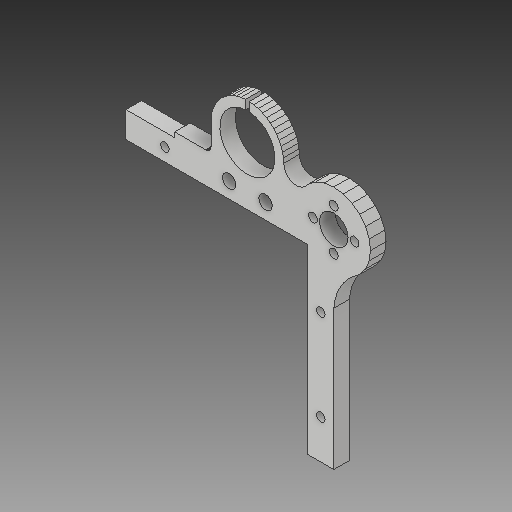
# Autodesk Inventor part: Left Bed Holder Mid
Saved by Autodesk Inventor 2017 (Build 210142000, 142)
## iProperties
Created: 2016-07-12
Part Number: Left Bed Holder Mid
Material: Generic
Document SubType Name: Modeling
Designer: joshmamo
Density: 1 g/cm^3
Appearance: Default
Author: joshmamo
Autodesk Inventor part; units mm, degrees
ref_plane "YZ Plane" through (0, 0, 0) normal (1, 0, 0) x (0, 1, 0)
ref_plane "XZ Plane" through (0, 0, 0) normal (0, 1, 0) x (-1, 0, 0)
ref_plane "XY Plane" through (0, 0, 0) normal (0, 0, 1) x (1, 0, 0)
sketch "Sketch1" plane through (0, 0, 0) normal (0, 0, 1) x (1, 0, 0)
  line L0 (-44.3097, 851.5953) -> (-45.3245, 852.187)
  line L1 (-39.0644, 849.737) -> (-39.5044, 849.6791)
  line L2 (-39.5044, 849.6791) -> (-39.9144, 849.5092)
  line L3 (-39.9144, 849.5092) -> (-40.2665, 849.2391)
  line L4 (-40.2665, 849.2391) -> (-40.5367, 848.887)
  line L5 (-40.5367, 848.887) -> (-40.7065, 848.477)
  line L6 (-40.7065, 848.477) -> (-40.7644, 848.037)
  line L7 (-40.7644, 848.037) -> (-40.7065, 847.597)
  line L8 (-40.7065, 847.597) -> (-40.5367, 847.187)
  line L9 (-40.5367, 847.187) -> (-40.2665, 846.8349)
  line L10 (-40.2665, 846.8349) -> (-39.9144, 846.5647)
  line L11 (-39.9144, 846.5647) -> (-39.5044, 846.3949)
  line L12 (-39.5044, 846.3949) -> (-39.0644, 846.337)
  line L13 (-39.0644, 846.337) -> (-38.6245, 846.3949)
  line L14 (-38.6245, 846.3949) -> (-38.2144, 846.5647)
  line L15 (-38.2144, 846.5647) -> (-37.8624, 846.8349)
  line L16 (-37.8624, 846.8349) -> (-37.5922, 847.187)
  line L17 (-37.5922, 847.187) -> (-37.4224, 847.597)
  line L18 (-37.4224, 847.597) -> (-37.3644, 848.037)
  line L19 (-37.3644, 848.037) -> (-37.4224, 848.477)
  line L20 (-37.4224, 848.477) -> (-37.5922, 848.887)
  line L21 (-37.5922, 848.887) -> (-37.8624, 849.2391)
  line L22 (-37.8624, 849.2391) -> (-38.2144, 849.5092)
  line L23 (-38.2144, 849.5092) -> (-38.6245, 849.6791)
  line L24 (-38.6245, 849.6791) -> (-39.0644, 849.737)
  line L25 (-55.0644, 846.337) -> (-54.6245, 846.3949)
  line L26 (-54.6245, 846.3949) -> (-54.2144, 846.5647)
  line L27 (-54.2144, 846.5647) -> (-53.8624, 846.8349)
  line L28 (-53.8624, 846.8349) -> (-53.5922, 847.187)
  line L29 (-53.5922, 847.187) -> (-53.4224, 847.597)
  line L30 (-53.4224, 847.597) -> (-53.3644, 848.037)
  line L31 (-53.3644, 848.037) -> (-53.4224, 848.477)
  line L32 (-53.4224, 848.477) -> (-53.5922, 848.887)
  line L33 (-53.5922, 848.887) -> (-53.8624, 849.2391)
  line L34 (-53.8624, 849.2391) -> (-54.2144, 849.5092)
  line L35 (-54.2144, 849.5092) -> (-54.6245, 849.6791)
  line L36 (-54.6245, 849.6791) -> (-55.0644, 849.737)
  line L37 (-55.0644, 849.737) -> (-55.5044, 849.6791)
  line L38 (-55.5044, 849.6791) -> (-55.9144, 849.5092)
  line L39 (-55.9144, 849.5092) -> (-56.2665, 849.2391)
  line L40 (-56.2665, 849.2391) -> (-56.5367, 848.887)
  line L41 (-56.5367, 848.887) -> (-56.7065, 848.477)
  line L42 (-56.7065, 848.477) -> (-56.7644, 848.037)
  line L43 (-56.7644, 848.037) -> (-56.7065, 847.597)
  line L44 (-56.7065, 847.597) -> (-56.5367, 847.187)
  line L45 (-56.5367, 847.187) -> (-56.2665, 846.8349)
  line L46 (-56.2665, 846.8349) -> (-55.9144, 846.5647)
  line L47 (-55.9144, 846.5647) -> (-55.5044, 846.3949)
  line L48 (-55.5044, 846.3949) -> (-55.0644, 846.337)
  line L49 (-45.3644, 840.037) -> (-45.4224, 840.477)
  line L50 (-45.4224, 840.477) -> (-45.5922, 840.887)
  line L51 (-45.5922, 840.887) -> (-45.8624, 841.2391)
  line L52 (-45.8624, 841.2391) -> (-46.2144, 841.5092)
  line L53 (-46.2144, 841.5092) -> (-46.6245, 841.6791)
  line L54 (-46.6245, 841.6791) -> (-47.0644, 841.737)
  line L55 (-47.0644, 841.737) -> (-47.5044, 841.6791)
  line L56 (-47.5044, 841.6791) -> (-47.9144, 841.5092)
  line L57 (-47.9144, 841.5092) -> (-48.2665, 841.2391)
  line L58 (-48.2665, 841.2391) -> (-48.5367, 840.887)
  line L59 (-48.5367, 840.887) -> (-48.7065, 840.477)
  line L60 (-48.7065, 840.477) -> (-48.7644, 840.037)
  line L61 (-48.7644, 840.037) -> (-48.7065, 839.597)
  line L62 (-48.7065, 839.597) -> (-48.5367, 839.187)
  line L63 (-48.5367, 839.187) -> (-48.2665, 838.8349)
  line L64 (-48.2665, 838.8349) -> (-47.9144, 838.5647)
  line L65 (-47.9144, 838.5647) -> (-47.5044, 838.3949)
  line L66 (-47.5044, 838.3949) -> (-47.0644, 838.337)
  line L67 (-47.0644, 838.337) -> (-46.6245, 838.3949)
  line L68 (-46.6245, 838.3949) -> (-46.2144, 838.5647)
  line L69 (-46.2144, 838.5647) -> (-45.8624, 838.8349)
  line L70 (-45.8624, 838.8349) -> (-45.5922, 839.187)
  line L71 (-45.5922, 839.187) -> (-45.4224, 839.597)
  line L72 (-45.4224, 839.597) -> (-45.3644, 840.037)
  line L73 (-48.7644, 856.037) -> (-48.7065, 855.597)
  line L74 (-48.7065, 855.597) -> (-48.5367, 855.187)
  line L75 (-48.5367, 855.187) -> (-48.2665, 854.8349)
  line L76 (-48.2665, 854.8349) -> (-47.9144, 854.5647)
  line L77 (-47.9144, 854.5647) -> (-47.5044, 854.3949)
  line L78 (-47.5044, 854.3949) -> (-47.0644, 854.337)
  line L79 (-47.0644, 854.337) -> (-46.6245, 854.3949)
  line L80 (-46.6245, 854.3949) -> (-46.2144, 854.5647)
  line L81 (-46.2144, 854.5647) -> (-45.8624, 854.8349)
  line L82 (-45.8624, 854.8349) -> (-45.5922, 855.187)
  line L83 (-45.5922, 855.187) -> (-45.4224, 855.597)
  line L84 (-45.4224, 855.597) -> (-45.3644, 856.037)
  line L85 (-45.3644, 856.037) -> (-45.4224, 856.477)
  line L86 (-45.4224, 856.477) -> (-45.5922, 856.887)
  line L87 (-45.5922, 856.887) -> (-45.8624, 857.2391)
  line L88 (-45.8624, 857.2391) -> (-46.2144, 857.5092)
  line L89 (-46.2144, 857.5092) -> (-46.6245, 857.6791)
  line L90 (-46.6245, 857.6791) -> (-47.0644, 857.737)
  line L91 (-47.0644, 857.737) -> (-47.5044, 857.6791)
  line L92 (-47.5044, 857.6791) -> (-47.9144, 857.5092)
  line L93 (-47.9144, 857.5092) -> (-48.2665, 857.2391)
  line L94 (-48.2665, 857.2391) -> (-48.5367, 856.887)
  line L95 (-48.5367, 856.887) -> (-48.7065, 856.477)
  line L96 (-48.7065, 856.477) -> (-48.7644, 856.037)
  line L97 (-52.4786, 816.4915) -> (-52.0644, 816.437)
  line L98 (-52.0644, 816.437) -> (-51.6503, 816.4915)
  line L99 (-51.6503, 816.4915) -> (-51.2644, 816.6513)
  line L100 (-51.2644, 816.6513) -> (-50.9331, 816.9056)
  line L101 (-50.9331, 816.9056) -> (-50.6788, 817.237)
  line L102 (-50.6788, 817.237) -> (-50.519, 817.6229)
  line L103 (-50.519, 817.6229) -> (-50.4644, 818.037)
  line L104 (-50.4644, 818.037) -> (-50.519, 818.4511)
  line L105 (-50.519, 818.4511) -> (-50.6788, 818.837)
  line L106 (-50.6788, 818.837) -> (-50.9331, 819.1683)
  line L107 (-50.9331, 819.1683) -> (-51.2644, 819.4226)
  line L108 (-51.2644, 819.4226) -> (-51.6503, 819.5825)
  line L109 (-51.6503, 819.5825) -> (-52.0644, 819.637)
  line L110 (-52.0644, 819.637) -> (-52.4786, 819.5825)
  line L111 (-52.4786, 819.5825) -> (-52.8644, 819.4226)
  line L112 (-52.8644, 819.4226) -> (-53.1958, 819.1683)
  line L113 (-53.1958, 819.1683) -> (-53.4501, 818.837)
  line L114 (-53.4501, 818.837) -> (-53.6099, 818.4511)
  line L115 (-53.6099, 818.4511) -> (-53.6644, 818.037)
  line L116 (-53.6644, 818.037) -> (-53.6099, 817.6229)
  line L117 (-53.6099, 817.6229) -> (-53.4501, 817.237)
  line L118 (-53.4501, 817.237) -> (-53.1958, 816.9056)
  line L119 (-53.1958, 816.9056) -> (-52.8644, 816.6513)
  line L120 (-52.8644, 816.6513) -> (-52.4786, 816.4915)
  line L121 (-113.6099, 843.4511) -> (-113.6644, 843.037)
  line L122 (-113.6644, 843.037) -> (-113.6099, 842.6229)
  line L123 (-113.6099, 842.6229) -> (-113.4501, 842.237)
  line L124 (-113.4501, 842.237) -> (-113.1958, 841.9056)
  line L125 (-113.1958, 841.9056) -> (-112.8644, 841.6513)
  line L126 (-112.8644, 841.6513) -> (-112.4786, 841.4915)
  line L127 (-112.4786, 841.4915) -> (-112.0644, 841.437)
  line L128 (-112.0644, 841.437) -> (-111.6503, 841.4915)
  line L129 (-111.6503, 841.4915) -> (-111.2644, 841.6513)
  line L130 (-111.2644, 841.6513) -> (-110.9331, 841.9056)
  line L131 (-110.9331, 841.9056) -> (-110.6788, 842.237)
  line L132 (-110.6788, 842.237) -> (-110.519, 842.6229)
  line L133 (-110.519, 842.6229) -> (-110.4644, 843.037)
  line L134 (-110.4644, 843.037) -> (-110.519, 843.4511)
  line L135 (-110.519, 843.4511) -> (-110.6788, 843.837)
  line L136 (-110.6788, 843.837) -> (-110.9331, 844.1683)
  line L137 (-110.9331, 844.1683) -> (-111.2644, 844.4226)
  line L138 (-111.2644, 844.4226) -> (-111.6503, 844.5825)
  line L139 (-111.6503, 844.5825) -> (-112.0644, 844.637)
  line L140 (-112.0644, 844.637) -> (-112.4786, 844.5825)
  line L141 (-112.4786, 844.5825) -> (-112.8644, 844.4226)
  line L142 (-112.8644, 844.4226) -> (-113.1958, 844.1683)
  line L143 (-113.1958, 844.1683) -> (-113.4501, 843.837)
  line L144 (-113.4501, 843.837) -> (-113.6099, 843.4511)
  line L145 (-52.4786, 781.4915) -> (-52.0644, 781.437)
  line L146 (-52.0644, 781.437) -> (-51.6503, 781.4915)
  line L147 (-51.6503, 781.4915) -> (-51.2644, 781.6513)
  line L148 (-51.2644, 781.6513) -> (-50.9331, 781.9056)
  line L149 (-50.9331, 781.9056) -> (-50.6788, 782.237)
  line L150 (-50.6788, 782.237) -> (-50.519, 782.6229)
  line L151 (-50.519, 782.6229) -> (-50.4644, 783.037)
  line L152 (-50.4644, 783.037) -> (-50.519, 783.4511)
  line L153 (-50.519, 783.4511) -> (-50.6788, 783.837)
  line L154 (-50.6788, 783.837) -> (-50.9331, 784.1683)
  line L155 (-50.9331, 784.1683) -> (-51.2644, 784.4226)
  line L156 (-51.2644, 784.4226) -> (-51.6503, 784.5825)
  line L157 (-51.6503, 784.5825) -> (-52.0644, 784.637)
  line L158 (-52.0644, 784.637) -> (-52.4786, 784.5825)
  line L159 (-52.4786, 784.5825) -> (-52.8644, 784.4226)
  line L160 (-52.8644, 784.4226) -> (-53.1958, 784.1683)
  line L161 (-53.1958, 784.1683) -> (-53.4501, 783.837)
  line L162 (-53.4501, 783.837) -> (-53.6099, 783.4511)
  line L163 (-53.6099, 783.4511) -> (-53.6644, 783.037)
  line L164 (-53.6644, 783.037) -> (-53.6099, 782.6229)
  line L165 (-53.6099, 782.6229) -> (-53.4501, 782.237)
  line L166 (-53.4501, 782.237) -> (-53.1958, 781.9056)
  line L167 (-53.1958, 781.9056) -> (-52.8644, 781.6513)
  line L168 (-52.8644, 781.6513) -> (-52.4786, 781.4915)
  line L169 (-127.0877, 838.0325) -> (-57.0877, 838.0325)
  line L170 (-57.0877, 838.0325) -> (-57.0877, 768.0325)
  line L171 (-57.0877, 768.0325) -> (-47.0644, 768.0325)
  line L172 (-47.0644, 768.0325) -> (-47.0644, 821.7992)
  arc A0 (-39.0184, 836.5858) -> (-47.0644, 821.7992) centre (-26.3948, 820.1343) ccw
  line L173 (-39.0184, 836.5858) -> (-37.0877, 838.0673)
  line L174 (-37.0877, 838.0673) -> (-34.8403, 840.9962)
  line L175 (-34.8403, 840.9962) -> (-33.4275, 844.407)
  line L176 (-33.4275, 844.407) -> (-32.9456, 848.0673)
  line L177 (-32.9456, 848.0673) -> (-33.4275, 851.7275)
  line L178 (-33.4275, 851.7275) -> (-34.8403, 855.1384)
  line L179 (-34.8403, 855.1384) -> (-37.0877, 858.0673)
  line L180 (-37.0877, 858.0673) -> (-40.0166, 860.3147)
  line L181 (-40.0166, 860.3147) -> (-43.4275, 861.7275)
  line L182 (-43.4275, 861.7275) -> (-47.0877, 862.2094)
  line L183 (-47.0877, 862.2094) -> (-50.748, 861.7275)
  line L184 (-50.748, 861.7275) -> (-54.1588, 860.3147)
  line L185 (-54.1588, 860.3147) -> (-57.0877, 858.0673)
  line L186 (-57.0877, 858.0673) -> (-57.9592, 856.9316)
  arc A1 (-66.3346, 860.4727) -> (-57.9592, 856.9316) centre (-61.3983, 860.4727) ccw
  line L187 (-66.3346, 860.4727) -> (-66.4468, 862.2422)
  line L188 (-66.4468, 862.2422) -> (-66.7819, 863.9833)
  line L189 (-66.7819, 863.9833) -> (-67.3343, 865.6681)
  line L190 (-67.3343, 865.6681) -> (-68.0952, 867.2696)
  line L191 (-68.0952, 867.2696) -> (-69.0524, 868.762)
  line L192 (-69.0524, 868.762) -> (-70.1906, 870.1215)
  line L193 (-70.1906, 870.1215) -> (-71.4915, 871.3262)
  line L194 (-71.4915, 871.3262) -> (-72.9342, 872.3569)
  line L195 (-72.9342, 872.3569) -> (-74.4956, 873.197)
  line L196 (-74.4956, 873.197) -> (-76.1507, 873.8329)
  line L197 (-76.1507, 873.8329) -> (-77.8729, 874.2546)
  line L198 (-77.8729, 874.2546) -> (-79.6346, 874.4552)
  line L199 (-79.6346, 874.4552) -> (-79.6346, 870.9493)
  line L200 (-79.6346, 870.9493) -> (-77.9981, 870.7094)
  line L201 (-77.9981, 870.7094) -> (-76.4195, 870.2155)
  line L202 (-76.4195, 870.2155) -> (-74.9382, 869.4798)
  line L203 (-74.9382, 869.4798) -> (-73.5907, 868.5207)
  line L204 (-73.5907, 868.5207) -> (-72.4106, 867.3618)
  line L205 (-72.4106, 867.3618) -> (-71.427, 866.032)
  line L206 (-71.427, 866.032) -> (-70.6646, 864.5643)
  line L207 (-70.6646, 864.5643) -> (-70.142, 862.995)
  line L208 (-70.142, 862.995) -> (-69.8724, 861.3631)
  line L209 (-69.8724, 861.3631) -> (-69.8623, 859.7092)
  line L210 (-69.8623, 859.7092) -> (-70.1122, 858.0742)
  line L211 (-70.1122, 858.0742) -> (-70.6156, 856.4987)
  line L212 (-70.6156, 856.4987) -> (-71.3603, 855.0218)
  line L213 (-71.3603, 855.0218) -> (-72.3276, 853.6801)
  line L214 (-72.3276, 853.6801) -> (-73.4936, 852.5071)
  line L215 (-73.4936, 852.5071) -> (-74.8293, 851.5316)
  line L216 (-74.8293, 851.5316) -> (-76.3017, 850.778)
  line L217 (-76.3017, 850.778) -> (-77.8741, 850.265)
  line L218 (-77.8741, 850.265) -> (-79.5076, 850.0053)
  line L219 (-79.5076, 850.0053) -> (-81.1615, 850.0053)
  line L220 (-81.1615, 850.0053) -> (-82.795, 850.265)
  line L221 (-82.795, 850.265) -> (-84.3674, 850.778)
  line L222 (-84.3674, 850.778) -> (-85.8398, 851.5316)
  line L223 (-85.8398, 851.5316) -> (-87.1755, 852.5071)
  line L224 (-87.1755, 852.5071) -> (-88.3415, 853.6801)
  line L225 (-88.3415, 853.6801) -> (-89.3088, 855.0218)
  line L226 (-89.3088, 855.0218) -> (-90.0535, 856.4987)
  line L227 (-90.0535, 856.4987) -> (-90.5569, 858.0742)
  line L228 (-90.5569, 858.0742) -> (-90.8068, 859.7092)
  line L229 (-90.8068, 859.7092) -> (-90.7967, 861.3631)
  line L230 (-90.7967, 861.3631) -> (-90.5271, 862.995)
  line L231 (-90.5271, 862.995) -> (-90.0046, 864.5643)
  line L232 (-90.0046, 864.5643) -> (-89.2421, 866.032)
  line L233 (-89.2421, 866.032) -> (-88.2586, 867.3618)
  line L234 (-88.2586, 867.3618) -> (-87.0784, 868.5207)
  line L235 (-87.0784, 868.5207) -> (-85.731, 869.4798)
  line L236 (-85.731, 869.4798) -> (-84.2496, 870.2155)
  line L237 (-84.2496, 870.2155) -> (-82.6711, 870.7094)
  line L238 (-82.6711, 870.7094) -> (-81.0346, 870.9493)
  line L239 (-81.0346, 870.9493) -> (-81.0346, 874.4552)
  line L240 (-81.0346, 874.4552) -> (-82.7962, 874.2546)
  line L241 (-82.7962, 874.2546) -> (-84.5184, 873.8329)
  line L242 (-84.5184, 873.8329) -> (-86.1735, 873.197)
  line L243 (-86.1735, 873.197) -> (-87.7349, 872.3569)
  line L244 (-87.7349, 872.3569) -> (-89.1776, 871.3262)
  line L245 (-89.1776, 871.3262) -> (-90.4785, 870.1215)
  line L246 (-90.4785, 870.1215) -> (-91.6167, 868.762)
  line L247 (-91.6167, 868.762) -> (-92.5739, 867.2696)
  line L248 (-92.5739, 867.2696) -> (-93.3349, 865.6681)
  line L249 (-93.3349, 865.6681) -> (-93.8873, 863.9833)
  line L250 (-93.8873, 863.9833) -> (-94.2223, 862.2422)
  line L251 (-94.2223, 862.2422) -> (-94.3346, 860.4727)
  line L252 (-94.3346, 860.4727) -> (-94.3346, 852.0727)
  line L253 (-94.3346, 852.0727) -> (-94.3665, 851.708)
  line L254 (-94.3665, 851.708) -> (-94.4612, 851.3544)
  line L255 (-94.4612, 851.3544) -> (-94.6159, 851.0227)
  line L256 (-94.6159, 851.0227) -> (-94.8259, 850.7228)
  line L257 (-94.8259, 850.7228) -> (-95.0847, 850.464)
  line L258 (-95.0847, 850.464) -> (-95.3846, 850.254)
  line L259 (-95.3846, 850.254) -> (-95.7163, 850.0993)
  line L260 (-95.7163, 850.0993) -> (-96.0699, 850.0046)
  line L261 (-96.0699, 850.0046) -> (-96.4346, 849.9727)
  line L262 (-96.4346, 849.9727) -> (-108.3345, 849.9727)
  line L263 (-108.3345, 849.9727) -> (-108.3345, 848.0325)
  line L264 (-108.3345, 848.0325) -> (-127.0877, 848.0325)
  line L265 (-127.0877, 848.0325) -> (-127.0877, 838.0325)
  line L266 (-127.0877, 838.0325) -> (-57.0877, 838.0325)
  line L267 (-57.0877, 838.0325) -> (-57.0877, 768.0325)
  line L268 (-57.0877, 768.0325) -> (-47.0644, 768.0325)
  line L269 (-47.0644, 768.0325) -> (-47.0644, 821.7992)
  arc A2 (-39.0184, 836.5858) -> (-47.0644, 821.7992) centre (-26.3948, 820.1343) ccw
  line L270 (-39.0184, 836.5858) -> (-37.0877, 838.0673)
  line L271 (-37.0877, 838.0673) -> (-34.8403, 840.9962)
  line L272 (-34.8403, 840.9962) -> (-33.4275, 844.407)
  line L273 (-33.4275, 844.407) -> (-32.9456, 848.0673)
  line L274 (-32.9456, 848.0673) -> (-33.4275, 851.7275)
  line L275 (-33.4275, 851.7275) -> (-34.8403, 855.1384)
  line L276 (-34.8403, 855.1384) -> (-37.0877, 858.0673)
  line L277 (-37.0877, 858.0673) -> (-40.0166, 860.3147)
  line L278 (-40.0166, 860.3147) -> (-43.4275, 861.7275)
  line L279 (-43.4275, 861.7275) -> (-47.0877, 862.2094)
  line L280 (-47.0877, 862.2094) -> (-50.748, 861.7275)
  line L281 (-50.748, 861.7275) -> (-54.1588, 860.3147)
  line L282 (-54.1588, 860.3147) -> (-57.0877, 858.0673)
  line L283 (-57.0877, 858.0673) -> (-57.9592, 856.9316)
  arc A3 (-66.3346, 860.4727) -> (-57.9592, 856.9316) centre (-61.3983, 860.4727) ccw
  line L284 (-66.3346, 860.4727) -> (-66.4468, 862.2422)
  line L285 (-66.4468, 862.2422) -> (-66.7819, 863.9833)
  line L286 (-66.7819, 863.9833) -> (-67.3343, 865.6681)
  line L287 (-67.3343, 865.6681) -> (-68.0952, 867.2696)
  line L288 (-68.0952, 867.2696) -> (-69.0524, 868.762)
  line L289 (-69.0524, 868.762) -> (-70.1906, 870.1215)
  line L290 (-70.1906, 870.1215) -> (-71.4915, 871.3262)
  line L291 (-71.4915, 871.3262) -> (-72.9342, 872.3569)
  line L292 (-72.9342, 872.3569) -> (-74.4956, 873.197)
  line L293 (-74.4956, 873.197) -> (-76.1507, 873.8329)
  line L294 (-76.1507, 873.8329) -> (-77.8729, 874.2546)
  line L295 (-77.8729, 874.2546) -> (-79.6346, 874.4552)
  line L296 (-79.6346, 874.4552) -> (-79.6346, 870.9493)
  line L297 (-79.6346, 870.9493) -> (-77.9981, 870.7094)
  line L298 (-77.9981, 870.7094) -> (-76.4195, 870.2155)
  line L299 (-76.4195, 870.2155) -> (-74.9382, 869.4798)
  line L300 (-74.9382, 869.4798) -> (-73.5907, 868.5207)
  line L301 (-73.5907, 868.5207) -> (-72.4106, 867.3618)
  line L302 (-72.4106, 867.3618) -> (-71.427, 866.032)
  line L303 (-71.427, 866.032) -> (-70.6646, 864.5643)
  line L304 (-70.6646, 864.5643) -> (-70.142, 862.995)
  line L305 (-70.142, 862.995) -> (-69.8724, 861.3631)
  line L306 (-69.8724, 861.3631) -> (-69.8623, 859.7092)
  line L307 (-69.8623, 859.7092) -> (-70.1122, 858.0742)
  line L308 (-70.1122, 858.0742) -> (-70.6156, 856.4987)
  line L309 (-70.6156, 856.4987) -> (-71.3603, 855.0218)
  line L310 (-71.3603, 855.0218) -> (-72.3276, 853.6801)
  line L311 (-72.3276, 853.6801) -> (-73.4936, 852.5071)
  line L312 (-73.4936, 852.5071) -> (-74.8293, 851.5316)
  line L313 (-74.8293, 851.5316) -> (-76.3017, 850.778)
  line L314 (-76.3017, 850.778) -> (-77.8741, 850.265)
  line L315 (-77.8741, 850.265) -> (-79.5076, 850.0053)
  line L316 (-79.5076, 850.0053) -> (-81.1615, 850.0053)
  line L317 (-81.1615, 850.0053) -> (-82.795, 850.265)
  line L318 (-82.795, 850.265) -> (-84.3674, 850.778)
  line L319 (-84.3674, 850.778) -> (-85.8398, 851.5316)
  line L320 (-85.8398, 851.5316) -> (-87.1755, 852.5071)
  line L321 (-87.1755, 852.5071) -> (-88.3415, 853.6801)
  line L322 (-88.3415, 853.6801) -> (-89.3088, 855.0218)
  line L323 (-89.3088, 855.0218) -> (-90.0535, 856.4987)
  line L324 (-90.0535, 856.4987) -> (-90.5569, 858.0742)
  line L325 (-90.5569, 858.0742) -> (-90.8068, 859.7092)
  line L326 (-90.8068, 859.7092) -> (-90.7967, 861.3631)
  line L327 (-90.7967, 861.3631) -> (-90.5271, 862.995)
  line L328 (-90.5271, 862.995) -> (-90.0046, 864.5643)
  line L329 (-90.0046, 864.5643) -> (-89.2421, 866.032)
  line L330 (-89.2421, 866.032) -> (-88.2586, 867.3618)
  line L331 (-88.2586, 867.3618) -> (-87.0784, 868.5207)
  line L332 (-87.0784, 868.5207) -> (-85.731, 869.4798)
  line L333 (-85.731, 869.4798) -> (-84.2496, 870.2155)
  line L334 (-84.2496, 870.2155) -> (-82.6711, 870.7094)
  line L335 (-82.6711, 870.7094) -> (-81.0346, 870.9493)
  line L336 (-81.0346, 870.9493) -> (-81.0346, 874.4552)
  line L337 (-81.0346, 874.4552) -> (-82.7962, 874.2546)
  line L338 (-82.7962, 874.2546) -> (-84.5184, 873.8329)
  line L339 (-84.5184, 873.8329) -> (-86.1735, 873.197)
  line L340 (-86.1735, 873.197) -> (-87.7349, 872.3569)
  line L341 (-87.7349, 872.3569) -> (-89.1776, 871.3262)
  line L342 (-89.1776, 871.3262) -> (-90.4785, 870.1215)
  line L343 (-90.4785, 870.1215) -> (-91.6167, 868.762)
  line L344 (-91.6167, 868.762) -> (-92.5739, 867.2696)
  line L345 (-92.5739, 867.2696) -> (-93.3349, 865.6681)
  line L346 (-93.3349, 865.6681) -> (-93.8873, 863.9833)
  line L347 (-93.8873, 863.9833) -> (-94.2223, 862.2422)
  line L348 (-94.2223, 862.2422) -> (-94.3346, 860.4727)
  line L349 (-94.3346, 860.4727) -> (-94.3346, 852.0727)
  line L350 (-94.3346, 852.0727) -> (-94.3665, 851.708)
  line L351 (-94.3665, 851.708) -> (-94.4612, 851.3544)
  line L352 (-94.4612, 851.3544) -> (-94.6159, 851.0227)
  line L353 (-94.6159, 851.0227) -> (-94.8259, 850.7228)
  line L354 (-94.8259, 850.7228) -> (-95.0847, 850.464)
  line L355 (-95.0847, 850.464) -> (-95.3846, 850.254)
  line L356 (-95.3846, 850.254) -> (-95.7163, 850.0993)
  line L357 (-95.7163, 850.0993) -> (-96.0699, 850.0046)
  line L358 (-96.0699, 850.0046) -> (-96.4346, 849.9727)
  line L359 (-96.4346, 849.9727) -> (-108.3345, 849.9727)
  line L360 (-108.3345, 849.9727) -> (-108.3345, 848.0325)
  line L361 (-108.3345, 848.0325) -> (-127.0877, 848.0325)
  line L362 (-127.0877, 848.0325) -> (-127.0877, 838.0325)
  line L363 (-57.0877, 768.0325) -> (-57.0877, 838.0325)
  line L364 (-57.0877, 838.0325) -> (-127.0877, 838.0325)
  line L365 (-57.0877, 838.0325) -> (-127.0877, 838.0325)
  line L366 (-57.0877, 768.0325) -> (-57.0877, 838.0325)
  line L367 (-127.0877, 848.0325) -> (-108.3345, 848.0325)
  line L368 (-108.3345, 848.0325) -> (-108.3345, 849.9727)
  line L369 (-108.3345, 849.9727) -> (-96.4346, 849.9727)
  line L370 (-96.4346, 849.9727) -> (-96.0699, 850.0046)
  line L371 (-96.0699, 850.0046) -> (-95.7163, 850.0993)
  line L372 (-95.7163, 850.0993) -> (-95.3846, 850.254)
  line L373 (-95.3846, 850.254) -> (-95.0847, 850.464)
  line L374 (-95.0847, 850.464) -> (-94.8259, 850.7228)
  line L375 (-94.8259, 850.7228) -> (-94.6159, 851.0227)
  line L376 (-94.6159, 851.0227) -> (-94.4612, 851.3544)
  line L377 (-94.4612, 851.3544) -> (-94.3665, 851.708)
  line L378 (-94.3665, 851.708) -> (-94.3346, 852.0727)
  line L379 (-94.3346, 852.0727) -> (-94.3346, 860.4727)
  line L380 (-94.3346, 860.4727) -> (-94.2223, 862.2422)
  line L381 (-94.2223, 862.2422) -> (-93.8873, 863.9833)
  line L382 (-93.8873, 863.9833) -> (-93.3349, 865.6681)
  line L383 (-93.3349, 865.6681) -> (-92.5739, 867.2696)
  line L384 (-92.5739, 867.2696) -> (-91.6167, 868.762)
  line L385 (-91.6167, 868.762) -> (-90.4785, 870.1215)
  line L386 (-90.4785, 870.1215) -> (-89.1776, 871.3262)
  line L387 (-89.1776, 871.3262) -> (-87.7349, 872.3569)
  line L388 (-87.7349, 872.3569) -> (-86.1735, 873.197)
  line L389 (-86.1735, 873.197) -> (-84.5184, 873.8329)
  line L390 (-84.5184, 873.8329) -> (-82.7962, 874.2546)
  line L391 (-82.7962, 874.2546) -> (-81.0346, 874.4552)
  line L392 (-81.0346, 874.4552) -> (-81.0346, 870.9493)
  line L393 (-81.0346, 870.9493) -> (-82.6711, 870.7094)
  line L394 (-82.6711, 870.7094) -> (-84.2496, 870.2155)
  line L395 (-84.2496, 870.2155) -> (-85.731, 869.4798)
  line L396 (-85.731, 869.4798) -> (-87.0784, 868.5207)
  line L397 (-87.0784, 868.5207) -> (-88.2586, 867.3618)
  line L398 (-88.2586, 867.3618) -> (-89.2421, 866.032)
  line L399 (-89.2421, 866.032) -> (-90.0046, 864.5643)
  line L400 (-90.0046, 864.5643) -> (-90.5271, 862.995)
  line L401 (-90.5271, 862.995) -> (-90.7967, 861.3631)
  line L402 (-90.7967, 861.3631) -> (-90.8068, 859.7092)
  line L403 (-90.8068, 859.7092) -> (-90.5569, 858.0742)
  line L404 (-90.5569, 858.0742) -> (-90.0535, 856.4987)
  line L405 (-90.0535, 856.4987) -> (-89.3088, 855.0218)
  line L406 (-89.3088, 855.0218) -> (-88.3415, 853.6801)
  line L407 (-88.3415, 853.6801) -> (-87.1755, 852.5071)
  line L408 (-87.1755, 852.5071) -> (-85.8398, 851.5316)
  line L409 (-85.8398, 851.5316) -> (-84.3674, 850.778)
  line L410 (-84.3674, 850.778) -> (-82.795, 850.265)
  line L411 (-82.795, 850.265) -> (-81.1615, 850.0053)
  line L412 (-81.1615, 850.0053) -> (-79.5076, 850.0053)
  line L413 (-79.5076, 850.0053) -> (-77.8741, 850.265)
  line L414 (-77.8741, 850.265) -> (-76.3017, 850.778)
  line L415 (-76.3017, 850.778) -> (-74.8293, 851.5316)
  line L416 (-74.8293, 851.5316) -> (-73.4936, 852.5071)
  line L417 (-73.4936, 852.5071) -> (-72.3276, 853.6801)
  line L418 (-72.3276, 853.6801) -> (-71.3603, 855.0218)
  line L419 (-71.3603, 855.0218) -> (-70.6156, 856.4987)
  line L420 (-70.6156, 856.4987) -> (-70.1122, 858.0742)
  line L421 (-70.1122, 858.0742) -> (-69.8623, 859.7092)
  line L422 (-69.8623, 859.7092) -> (-69.8724, 861.3631)
  line L423 (-69.8724, 861.3631) -> (-70.142, 862.995)
  line L424 (-70.142, 862.995) -> (-70.6646, 864.5643)
  line L425 (-70.6646, 864.5643) -> (-71.427, 866.032)
  line L426 (-71.427, 866.032) -> (-72.4106, 867.3618)
  line L427 (-72.4106, 867.3618) -> (-73.5907, 868.5207)
  line L428 (-73.5907, 868.5207) -> (-74.9382, 869.4798)
  line L429 (-74.9382, 869.4798) -> (-76.4195, 870.2155)
  line L430 (-76.4195, 870.2155) -> (-77.9981, 870.7094)
  line L431 (-77.9981, 870.7094) -> (-79.6346, 870.9493)
  line L432 (-79.6346, 870.9493) -> (-79.6346, 874.4552)
  line L433 (-79.6346, 874.4552) -> (-77.8729, 874.2546)
  line L434 (-77.8729, 874.2546) -> (-76.1507, 873.8329)
  line L435 (-76.1507, 873.8329) -> (-74.4956, 873.197)
  line L436 (-74.4956, 873.197) -> (-72.9342, 872.3569)
  line L437 (-72.9342, 872.3569) -> (-71.4915, 871.3262)
  line L438 (-71.4915, 871.3262) -> (-70.1906, 870.1215)
  line L439 (-70.1906, 870.1215) -> (-69.0524, 868.762)
  line L440 (-69.0524, 868.762) -> (-68.0952, 867.2696)
  line L441 (-68.0952, 867.2696) -> (-67.3343, 865.6681)
  line L442 (-67.3343, 865.6681) -> (-66.7819, 863.9833)
  line L443 (-66.7819, 863.9833) -> (-66.4468, 862.2422)
  line L444 (-66.4468, 862.2422) -> (-66.3346, 860.4727)
  arc A4 (-66.3346, 860.4727) -> (-57.9592, 856.9316) centre (-61.3983, 860.4727) ccw
  line L445 (-57.9592, 856.9316) -> (-57.0877, 858.0673)
  line L446 (-57.0877, 858.0673) -> (-54.1588, 860.3147)
  line L447 (-54.1588, 860.3147) -> (-50.748, 861.7275)
  line L448 (-50.748, 861.7275) -> (-47.0877, 862.2094)
  line L449 (-47.0877, 862.2094) -> (-43.4275, 861.7275)
  line L450 (-43.4275, 861.7275) -> (-40.0166, 860.3147)
  line L451 (-40.0166, 860.3147) -> (-37.0877, 858.0673)
  line L452 (-37.0877, 858.0673) -> (-34.8403, 855.1384)
  line L453 (-34.8403, 855.1384) -> (-33.4275, 851.7275)
  line L454 (-33.4275, 851.7275) -> (-32.9456, 848.0673)
  line L455 (-32.9456, 848.0673) -> (-33.4275, 844.407)
  line L456 (-33.4275, 844.407) -> (-34.8403, 840.9962)
  line L457 (-34.8403, 840.9962) -> (-37.0877, 838.0673)
  line L458 (-37.0877, 838.0673) -> (-39.0184, 836.5858)
  arc A5 (-39.0184, 836.5858) -> (-47.0644, 821.7992) centre (-26.3948, 820.1343) ccw
  line L459 (-47.0644, 821.7992) -> (-47.0644, 768.0325)
  line L460 (-47.0644, 768.0325) -> (-57.0877, 768.0325)
  line L461 (-127.0877, 838.0325) -> (-127.0877, 848.0325)
  circle A6 centre (-47.0644, 848.0558) radius 5.5
  circle A7 centre (-87.3346, 844.0325) radius 2.6
  circle A8 centre (-73.3346, 844.0325) radius 2.6
  point P0 (0, 0)
  constraints: 924 end point, 12 point on circle, 9 centre point
extrude "Extrusion1" add sketch "Sketch1" along normal blind 6
sketch "Sketch2" plane through (0, 0, 0) normal (0, 0, -1) x (-1, 0, 0)
  line L0 (52.0644, 781.437) -> (52.4786, 781.4915) projected
  line L1 (52.0644, 784.637) -> (52.0644, 781.437)
  line L2 (51.6503, 819.5825) -> (52.0644, 819.637) projected
  line L3 (52.4786, 816.4915) -> (52.0644, 816.437) projected
  line L4 (52.0644, 819.637) -> (52.0644, 816.437)
  line L5 (112.4786, 844.5825) -> (112.0644, 844.637) projected
  line L6 (112.0644, 844.637) -> (112.0644, 841.437)
  line L7 (47.5044, 841.6791) -> (47.0644, 841.737) projected
  line L8 (47.0644, 838.337) -> (47.5044, 838.3949) projected
  line L9 (47.0644, 841.737) -> (47.0644, 838.337)
  line L10 (55.0644, 849.737) -> (54.6245, 849.6791) projected
  line L11 (55.0644, 849.737) -> (55.0644, 846.337)
  line L12 (47.0644, 857.737) -> (47.0644, 854.337)
  line L13 (39.0644, 849.737) -> (38.6245, 849.6791) projected
  line L14 (39.0644, 849.737) -> (39.0644, 846.337)
  point P0 (0, 0)
  point P1 (39.0644, 848.037)
  point P2 (47.0644, 856.037)
  point P3 (55.0644, 848.037)
  point P4 (47.0644, 840.037)
  point P5 (52.0644, 818.037)
  point P6 (52.0644, 783.037)
  point P7 (112.0644, 843.037)
  constraints: 14 end point, 7 midpoint, 7 vertical
hole "Hole1" at (-39.0644, 848.037, 0) at (-47.0644, 856.037, 0) at (-55.0644, 848.037, 0) at (-47.0644, 840.037, 0) at (-52.0644, 818.037, 0) at (-52.0644, 783.037, 0) at (-112.0644, 843.037, 0) direction (0, 0, 1) diameter 3.3 depth 8 tip angle 118
sketch "Sketch3" plane through (0, 0, 0) normal (0, 0, -1) x (-1, 0, 0)
  line L0 (46.6245, 838.3949) -> (47.0644, 838.337) projected
  line L1 (47.0644, 838.337) -> (47.0644, 841.737)
  line L2 (55.0644, 846.337) -> (55.5044, 846.3949) projected
  line L3 (55.5044, 849.6791) -> (55.0644, 849.737) projected
  line L4 (55.0644, 846.337) -> (55.0644, 849.737)
  line L5 (47.0644, 854.337) -> (47.5044, 854.3949) projected
  line L6 (47.0644, 854.337) -> (47.0644, 857.737)
  line L7 (39.5044, 846.3949) -> (39.0644, 846.337) projected
  line L8 (39.0644, 846.337) -> (39.0644, 849.737)
  point P0 (0, 0)
  point P1 (47.0644, 856.037)
  point P2 (55.0644, 848.037)
  point P3 (47.0644, 840.037)
  point P4 (39.0644, 848.037)
  constraints: 8 end point, 4 midpoint, 4 vertical
hole "Hole2" at (-47.0644, 856.037, 0) at (-55.0644, 848.037, 0) at (-47.0644, 840.037, 0) at (-39.0644, 848.037, 0) direction (0, 0, 1) diameter 3.4 depth 8 tip angle 118
sketch "Sketch4" plane through (0, 0, 0) normal (0, 0, -1) x (-1, 0, 0)
  arc A0 (79.6346, 870.9864) -> (81.0346, 870.9864) centre (80.3346, 860.4095) ccw
  point P0 (0, 0)
  constraints: 2 point on circle, 1 centre point
hole "Hole3" at (-80.3346, 860.4095, 0) direction (0, 0, 1) diameter 21.2 depth 8 tip angle 118
body "Solid1"
